# Autodesk Inventor part: 2_2U
Saved by Autodesk Inventor 2016 (Build 200138000, 138)
## iProperties
Created: 2016-04-08
Part Number: 2_2U
Material: Generic
Document SubType Name: Modeling
Designer: Paschalis
Density: 1 g/cm^3
Appearance: C3216, 2_2U
Author: Paschalis
Autodesk Inventor part; units mm, degrees
ref_plane "YZ Plane" through (0, 0, 0) normal (1, 0, 0) x (0, 1, 0)
ref_plane "XZ Plane" through (0, 0, 0) normal (0, 1, 0) x (-1, 0, 0)
ref_plane "XY Plane" through (0, 0, 0) normal (0, 0, 1) x (1, 0, 0)
sketch "C3216, 2_2U_51" plane through (0, 0, 0) normal (0, 0, 1) x (1, 0, 0)
  line L0 (-2.4984, 1.0084) -> (2.4984, 1.0084)
  line L1 (2.4984, 1.0084) -> (2.4984, -0.983)
  line L2 (2.4984, -0.983) -> (-2.4984, -0.983)
  line L3 (-2.4984, -0.983) -> (-2.4984, 1.0084)
  constraints: 8 end point
extrude "Extrusion1" add sketch "C3216, 2_2U_51" along normal blind 1
body "Solid1"
